small_button (Autodesk Fusion 360 design; units mm, degrees)
Autodesk Fusion 360 part; units mm, degrees
sketch "Sketch1" plane through (0, 0, 0) normal (0, 1, 0) x (1, 0, 0)
  line L0 (0, 0) -> (-7, 0)
  line L1 (-7, 0) -> (-7, -7)
  line L2 (-7, -7) -> (0, -7)
  line L3 (0, -7) -> (0, 0)
  dimension "d1" = 7
  dimension "d2" = 7
  constraint horizontal L0
  constraint vertical L1
  constraint horizontal L2
  constraint vertical L3
  constraint coincident L0.start L3.end
  measures "d1" distance of L1.end L2.end
  measures "d2" distance of L0.end L1.end
extrude "Extrude1" add sketch "Sketch1" along normal blind 4
sketch "Sketch2" plane through (0, 4, 0) normal (0, 1, 0) x (-1, 0, 0)
  line L0 (0, 7) -> (0, 0)
  line L1 (0, 0) -> (7, 0)
  line L2 (7, 0) -> (7, 7)
  line L3 (7, 7) -> (0, 7)
  line L4 (3.5, 7) -> (3.5, 0)
  line L5 (7, 3.5) -> (0, 3.5)
  circle A0 centre (3.5, 3.5) radius 1.7
  dimension "d5" = 3.4
  constraint midpoint L3 L4.start
  constraint midpoint L1 L4.end
  constraint midpoint L2 L5.start
  constraint midpoint L0 L5.end
  constraint midpoint L5 A0.centre
  measures "d5" diameter of A0
extrude "Extrude2" add sketch "Sketch2" along normal blind 8.7 contours L4 L5 A0 | L4 L5 A0 | L4 L5 A0 | L4 L5 A0
ref_plane "WorkPlane1" through (-3.5, 0, 0) normal (1, 0, 0) x (0, 1, 0)
sketch "Sketch3" plane through (0, 0, 0) normal (1, 0, 0) x (0, 1, 0)
  line L0 (0, 7) -> (0, 0)
  line L1 (0, 0) -> (4, 0)
  line L2 (4, 0) -> (4, 7)
  line L3 (4, 7) -> (0, 7)
  line L4 (2.5, 0) -> (-1, 0)
  line L5 (-1, 0) -> (-1, 1.9)
  line L6 (-1, 1.9) -> (2.5, 1.9)
  line L7 (2.5, 1.9) -> (2.5, 0)
  line L8 (2.5, 7) -> (-1, 7)
  line L9 (-1, 7) -> (-1, 5.1)
  line L10 (-1, 5.1) -> (2.5, 5.1)
  line L11 (2.5, 5.1) -> (2.5, 7)
  line L12 (4, 7) -> (4, 0)
  dimension "d9" = 1.9
  dimension "d10" = 1.9
  dimension "d11" = 1.5
  dimension "d12" = 1.5
  dimension "d13" = 3.5
  dimension "d14" = 3.5
  constraint horizontal L4
  constraint vertical L5
  constraint horizontal L6
  constraint vertical L7
  constraint coincident L1 L4.start
  constraint horizontal L8
  constraint vertical L9
  constraint horizontal L10
  constraint vertical L11
  constraint coincident L3 L8.start
  measures "d9" distance of L4.start L6.end
  measures "d10" distance of L8.start L10.end
  measures "d11" distance of L7 L12
  measures "d12" distance of L11 L12
  measures "d13" distance of L4.start L4.end
  measures "d14" distance of L8.start L8.end
extrude "Extrude3" add sketch "Sketch3" along normal blind 1.6 contours L0 L3 L8 L10 L11 | L0 L8 L9 L10 | L0 L1 L4 L6 L7 | L0 L4 L5 L6
mirror "Mirror1" about plane through (-3.5, 0, 0) normal (1, 0, 0) of "Extrude3"
equation "d2 = d1"
equation "d10 = d9"
equation "d12 = d11"
equation "d14 = d13"
